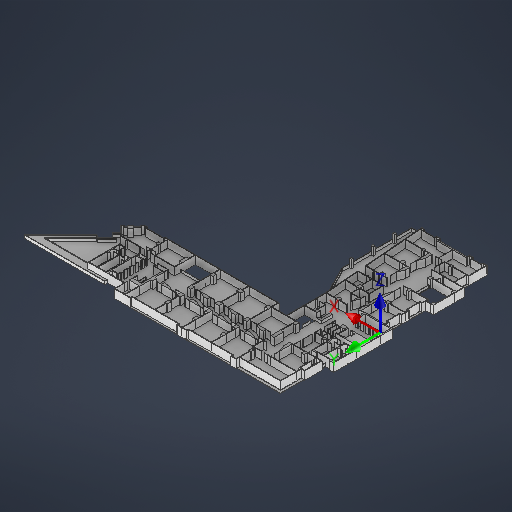
# Autodesk Inventor part: CIT-Floor-6
Saved by Autodesk Inventor 2026.1 (Build 301233020, 233B)
## iProperties
Created: 2025-08-04
Part Number: CIT-Floor-6
Material: Generic
Document SubType Name: Modeling
Designer: diego
Density: 1 g/cm^3
Appearance: Default
Author: diego
Autodesk Inventor part; units mm, degrees
(part 1 of 2)
ref_plane "YZ Plane" through (0, 0, 0) normal (1, 0, 0) x (0, 1, 0)
ref_plane "XZ Plane" through (0, 0, 0) normal (0, 1, 0) x (-1, 0, 0)
ref_plane "XY Plane" through (0, 0, 0) normal (0, 0, 1) x (1, 0, 0)
sketch "Architecture" plane through (0, 0, 0) normal (0, 1, 0) x (-1, 0, 0)
  line L0 (-168175.668, 0) -> (0, 0) construction
  line L1 (0, 0) -> (0, -118792.8893) construction
  line L2 (0, -118792.8893) -> (-168175.668, -118792.8893) construction
  line L3 (-168175.668, -118792.8893) -> (-168175.668, 0) construction
  line L4 (-25977.9567, -19239.0056) -> (-38827.9567, -19239.0056) construction
  line L5 (-23543, -30793.9912) -> (-42293, -30793.9912)
  line L6 (-42293, -30793.9912) -> (-42293, -44243.9912)
  line L7 (-42293, -44243.9912) -> (-39853, -44243.9912)
  line L8 (-39853, -44243.9912) -> (-37304.8036, -46801.098)
  line L9 (-37304.8036, -46801.098) -> (-35746.456, -45248.1806)
  line L10 (-35040.5844, -45956.5204) -> (-36598.9321, -47509.4379)
  line L11 (-36598.9321, -47509.4379) -> (-36257.3538, -47852.2105)
  line L12 (-23543, -30793.9912) -> (-33652.9783, -40945.5475)
  line L13 (-33652.9783, -40945.5475) -> (-33794.1526, -40803.8796)
  line L14 (-33794.1526, -40803.8796) -> (-33935.8206, -40945.0539)
  line L15 (-33935.8206, -40945.0539) -> (-34281.6976, -40597.9673)
  line L16 (-34281.6976, -40597.9673) -> (-38106.7328, -44409.6738)
  line L17 (-38106.7328, -44409.6738) -> (-37577.3291, -44940.9287)
  line L18 (-35040.5844, -45956.5204) -> (-36812.3221, -44178.5874)
  line L19 (-42293, -30653.9912) -> (-42293, -28903.9912)
  line L20 (-37577.3291, -44940.9287) -> (-33752.294, -41129.2222)
  line L21 (-42293, -30653.9912) -> (-23205.9885, -30653.9912)
  line L22 (-18318.5941, -27753.9912) -> (-50017.455, -27753.9912)
  line L23 (-50017.455, -27753.9912) -> (-50017.455, -28903.9912)
  line L24 (-42293, -43593.9912) -> (-42573, -43593.9912)
  line L25 (-42293, -41543.9912) -> (-42573, -41543.9912)
  line L26 (-42573, -43593.9912) -> (-42573, -44243.9912)
  line L27 (-42573, -41543.9912) -> (-42573, -41363.9912)
  line L28 (-42573, -44243.9912) -> (-47323, -44243.9912)
  line L29 (-42573, -41363.9912) -> (-44583, -41363.9912)
  line L30 (-44583, -41363.9912) -> (-44583, -39763.9912)
  line L31 (-44583, -39763.9912) -> (-44433, -39763.9912)
  line L32 (-44433, -39763.9912) -> (-44433, -41133.9912)
  line L33 (-44583, -38763.9912) -> (-44583, -38623.9912)
  line L34 (-44583, -38623.9912) -> (-43788.5906, -38623.9912)
  line L35 (-44583, -38763.9912) -> (-42573, -38763.9912)
  line L36 (-44433, -41133.9912) -> (-42573, -41133.9912)
  line L37 (-42573, -41133.9912) -> (-42573, -38763.9912)
  line L38 (-42573, -36263.9912) -> (-42573, -29203.9912)
  line L39 (-43788.5906, -37583.9912) -> (-48088.5906, -37583.9912)
  line L40 (-48088.5906, -37583.9912) -> (-48088.5906, -37443.9912)
  line L41 (-43788.5906, -37443.9912) -> (-45798.5906, -37443.9912)
  line L42 (-45798.5906, -37443.9912) -> (-45798.5906, -29203.9912)
  line L43 (-48088.5906, -37443.9912) -> (-46078.5906, -37443.9912)
  line L44 (-46078.5906, -37443.9912) -> (-46078.5906, -29203.9912)
  line L45 (-43788.5906, -36403.9912) -> (-43788.5906, -36263.9912)
  line L46 (-43788.5906, -36263.9912) -> (-42573, -36263.9912)
  line L47 (-43788.5906, -36403.9912) -> (-43788.5906, -36403.9912)
  line L48 (-42293, -28903.9912) -> (-49867.455, -28903.9912)
  line L49 (-18667.455, -27903.9912) -> (-49867.455, -27903.9912)
  line L50 (-49867.455, -27903.9912) -> (-49867.455, -28903.9912)
  line L51 (-23205.9885, -30653.9912) -> (-33554.1556, -41044.7158)
  line L52 (-33554.1556, -41044.7158) -> (-32707.1097, -41894.7236)
  line L53 (-33752.294, -41129.2222) -> (-32749.9556, -42135.0655)
  line L54 (-32749.9556, -42135.0655) -> (-18318.5941, -27753.9912)
  line L55 (-32707.1097, -41894.7236) -> (-18667.455, -27903.9912)
  line L56 (-47033, -38763.9912) -> (-49453, -38763.9912)
  line L57 (-47033, -38763.9912) -> (-47033, -38623.9912)
  line L58 (-47033, -38623.9912) -> (-48088.5906, -38623.9912)
  line L59 (-48088.5906, -36403.9912) -> (-48088.5906, -36263.9912)
  line L60 (-48088.5906, -36263.9912) -> (-49453, -36263.9912)
  line L61 (-43788.5906, -37583.9912) -> (-43788.5906, -37443.9912)
  line L62 (-49453, -29203.9912) -> (-49453, -36263.9912)
  line L63 (-49453, -38763.9912) -> (-49453, -42193.9912)
  arc A0 (-43788.5906, -38623.9912) -> (-43788.5906, -36403.9912) centre (-43788.5906, -37513.9912) ccw
  line L64 (-49453, -42193.9912) -> (-52313, -42193.9912)
  line L65 (-47323, -44243.9912) -> (-47323, -44318.9912)
  line L66 (-47323, -44318.9912) -> (-49023, -44318.9912)
  line L67 (-49023, -44318.9912) -> (-49023, -44418.9912)
  line L68 (-49023, -44418.9912) -> (-47323, -44418.9912)
  line L69 (-47323, -44418.9912) -> (-47323, -44493.9912)
  line L70 (-50223, -45658.9912) -> (-50223, -44243.9912)
  line L71 (-50223, -44243.9912) -> (-50323, -44243.9912)
  line L72 (-50323, -44243.9912) -> (-50323, -45658.9912)
  line L73 (-47323, -44493.9912) -> (-39985, -44493.9912)
  line L74 (-39985, -44493.9912) -> (-36625.0513, -47865.6888)
  line L75 (-50223, -45658.9912) -> (-48423, -45658.9912)
  line L76 (-48423, -45658.9912) -> (-48423, -45758.9912)
  line L77 (-48423, -45758.9912) -> (-50223, -45758.9912)
  line L78 (-51523, -44318.9912) -> (-51523, -44418.9912)
  line L79 (-51523, -44418.9912) -> (-53223, -44418.9912)
  line L80 (-53223, -44418.9912) -> (-53223, -44493.9912)
  line L81 (-53223, -44493.9912) -> (-60843, -44493.9912)
  line L82 (-51523, -44318.9912) -> (-53223, -44318.9912)
  line L83 (-53223, -44318.9912) -> (-53223, -44243.9912)
  line L84 (-53223, -44243.9912) -> (-61093, -44243.9912)
  line L85 (-50323, -45658.9912) -> (-52123, -45658.9912)
  line L86 (-52123, -45658.9912) -> (-52123, -45758.9912)
  line L87 (-52123, -45758.9912) -> (-50323, -45758.9912)
  line L88 (-50323, -45758.9912) -> (-50323, -52377.8595)
  line L89 (-52313, -42193.9912) -> (-52313, -41883.9912)
  line L90 (-52313, -41883.9912) -> (-52163, -41883.9912)
  line L91 (-52163, -41883.9912) -> (-52163, -42042.9956)
  line L92 (-52163, -42042.9956) -> (-49603, -42042.9956)
  line L93 (-49603, -42042.9956) -> (-49603, -40973.9912)
  line L94 (-49603, -40973.9912) -> (-52313, -40973.9912)
  line L95 (-52313, -40973.9912) -> (-52313, -39823.9912)
  line L96 (-52313, -39823.9912) -> (-52113, -39823.9912)
  line L97 (-52113, -39823.9912) -> (-52113, -40474.0396)
  line L98 (-52113, -40474.0396) -> (-49603, -40474.0396)
  line L99 (-49603, -40474.0396) -> (-49603, -30963.9912)
  line L100 (-52313, -38803.9912) -> (-52313, -37793.9912)
  line L101 (-52313, -37793.9912) -> (-52113, -37793.9912)
  line L102 (-52113, -37793.9912) -> (-52113, -38803.9912)
  line L103 (-52113, -38803.9912) -> (-52313, -38803.9912)
  line L104 (-52113, -36773.9912) -> (-52313, -36773.9912)
  line L105 (-52313, -36773.9912) -> (-52313, -35493.9912)
  line L106 (-52313, -35493.9912) -> (-52113, -35493.9912)
  line L107 (-52113, -35493.9912) -> (-52113, -36773.9912)
  line L108 (-52113, -33153.9912) -> (-52313, -33153.9912)
  line L109 (-52313, -33153.9912) -> (-52313, -34473.9912)
  line L110 (-52313, -34473.9912) -> (-52113, -34473.9912)
  line L111 (-52113, -34473.9912) -> (-52113, -33153.9912)
  line L112 (-52113, -32133.9912) -> (-52313, -32133.9912)
  line L113 (-52313, -32133.9912) -> (-52313, -31613.9912)
  line L114 (-52113, -30963.9912) -> (-52113, -32133.9912)
  line L115 (-52313, -31613.9912) -> (-52373, -31613.9912)
  line L116 (-52373, -31613.9912) -> (-52373, -30963.9912)
  line L117 (-52373, -30963.9912) -> (-52313, -30963.9912)
  line L118 (-52313, -30963.9912) -> (-52313, -30163.9912)
  line L119 (-52313, -30163.9912) -> (-52163, -30163.9912)
  line L120 (-52163, -30163.9912) -> (-52163, -30663.9912)
  line L121 (-52163, -29203.9912) -> (-50078, -29203.9912)
  line L122 (-52163, -29203.9912) -> (-52163, -29253.9912)
  line L123 (-52163, -29253.9912) -> (-52313, -29253.9912)
  line L124 (-52313, -29253.9912) -> (-52313, -29203.9912)
  line L125 (-52313, -29203.9912) -> (-56513, -29203.9912)
  line L126 (-50017.455, -28903.9912) -> (-56513, -28903.9912)
  line L127 (-49603, -30963.9912) -> (-52113, -30963.9912)
  line L128 (-52163, -30663.9912) -> (-50078, -30663.9912)
  line L129 (-50078, -30663.9912) -> (-50078, -29203.9912)
  line L130 (-56513, -29203.9912) -> (-56513, -30003.9912)
  line L131 (-56513, -30003.9912) -> (-56663, -30003.9912)
  line L132 (-56663, -30003.9912) -> (-56663, -25231.5979)
  line L133 (-56513, -31613.9912) -> (-56513, -33963.9912)
  line L134 (-56453, -30963.9912) -> (-56453, -31613.9912)
  line L135 (-56453, -31613.9912) -> (-56513, -31613.9912)
  line L136 (-56453, -30963.9912) -> (-56513, -30963.9912)
  line L137 (-56513, -30963.9912) -> (-56513, -30913.9912)
  line L138 (-56513, -30913.9912) -> (-60463, -30913.9912)
  line L139 (-56513, -33963.9912) -> (-56763, -33963.9912)
  line L140 (-56763, -33963.9912) -> (-56763, -32263.9912)
  line L141 (-56763, -32263.9912) -> (-60063, -32263.9912)
  line L142 (-56513, -40463.9912) -> (-56513, -41093.9912)
  line L143 (-56513, -40463.9912) -> (-60063, -40463.9912)
  line L144 (-56513, -42043.9912) -> (-56513, -42193.9912)
  line L145 (-56513, -42043.9912) -> (-60563, -42043.9912)
  line L146 (-56513, -41093.9912) -> (-56663, -41093.9912)
  line L147 (-56513, -42193.9912) -> (-60713, -42193.9912)
  line L148 (-60063, -40463.9912) -> (-60063, -32263.9912)
  line L149 (-56663, -25231.5979) -> (-60463, -25231.5979)
  line L150 (-60463, -25231.5979) -> (-60463, -30913.9912)
  line L151 (-56513, -28903.9912) -> (-56513, -24981.5979)
  line L152 (-56513, -24981.5979) -> (-104613, -24981.5979)
  line L153 (-56638, -37333.9912) -> (-58388, -37333.9912)
  line L154 (-58388, -37333.9912) -> (-58388, -37033.9912)
  line L155 (-58388, -37033.9912) -> (-60063, -37033.9912)
  line L156 (-56638, -33963.9912) -> (-56638, -37333.9912)
  line L157 (-60713, -25231.5979) -> (-62573, -25231.5979)
  line L158 (-56663, -41093.9912) -> (-56663, -40613.9912)
  line L159 (-56663, -40613.9912) -> (-60563, -40613.9912)
  line L160 (-60563, -40613.9912) -> (-60563, -42043.9912)
  line L161 (-60843, -44493.9912) -> (-60843, -47343.9912)
  line L162 (-36257.3538, -47852.2105) -> (-41049.7021, -52627.8595)
  line L163 (-41049.7021, -52627.8595) -> (-93819.593, -52627.8595)
  line L164 (-36625.0513, -47865.6888) -> (-37050.0552, -48289.2118)
  line L165 (-37050.0552, -48289.2118) -> (-37402.991, -47935.0419)
  line L166 (-37402.991, -47935.0419) -> (-38199.8733, -48729.1474)
  line L167 (-38199.8733, -48729.1474) -> (-38834.9879, -48091.812)
  line L168 (-38834.9879, -48091.812) -> (-39954.1648, -49207.0891)
  line L169 (-39954.1648, -49207.0891) -> (-39319.0503, -49844.4245)
  line L170 (-39319.0503, -49844.4245) -> (-40948.2319, -51467.9291)
  line L171 (-40948.2319, -51467.9291) -> (-40595.2961, -51822.099)
  line L172 (-40595.2961, -51822.099) -> (-41153, -52377.8595)
  line L173 (-41153, -52377.8595) -> (-41873, -52377.8595)
  line L174 (-41873, -52377.8595) -> (-41873, -51877.8595)
  line L175 (-41873, -51877.8595) -> (-49073, -51877.8595)
  line L176 (-49073, -51877.8595) -> (-49073, -52377.8595)
  line L177 (-49073, -52377.8595) -> (-50223, -52377.8595)
  line L178 (-37050.6723, -48642.7646) -> (-37438.9017, -48253.1777)
  line L179 (-37438.9017, -48253.1777) -> (-38058.699, -48870.8153)
  line L180 (-38058.699, -48870.8153) -> (-37670.4697, -49260.4023)
  line L181 (-50323, -52377.8595) -> (-60843, -52377.8595)
  line L182 (-60843, -52377.8595) -> (-60843, -49993.9912)
  line L183 (-60843, -47343.9912) -> (-59923, -47343.9912)
  line L184 (-59923, -47343.9912) -> (-59923, -49993.9912)
  line L185 (-59923, -49993.9912) -> (-60843, -49993.9912)
  line L186 (-50223, -48728.9912) -> (-49263, -48728.9912)
  line L187 (-49263, -48728.9912) -> (-49263, -49689)
  line L188 (-49263, -49689) -> (-50223, -49689)
  line L189 (-50223, -45758.9912) -> (-50223, -48728.9912)
  line L190 (-50223, -49689) -> (-50223, -52377.8595)
  line L191 (-61093, -46693.9912) -> (-70593, -46693.9912)
  line L192 (-61093, -46793.9912) -> (-70593, -46793.9912)
  line L193 (-61093, -44243.9912) -> (-61093, -46693.9912)
  line L194 (-70593, -46693.9912) -> (-70593, -43483.9912)
  line L195 (-70593, -43483.9912) -> (-70443, -43483.9912)
  line L196 (-70443, -43483.9912) -> (-70443, -39883.9912)
  line L197 (-70443, -39883.9912) -> (-71793, -39883.9912)
  line L198 (-46078.5906, -29203.9912) -> (-49453, -29203.9912)
  line L199 (-45798.5906, -29203.9912) -> (-42573, -29203.9912)
  line L200 (-60713, -36893.9912) -> (-61393, -36893.9912)
  line L201 (-61393, -36893.9912) -> (-61393, -35293.9912)
  line L202 (-62613, -35843.9912) -> (-64413, -35843.9912)
  line L203 (-64413, -35843.9912) -> (-64413, -36893.9912)
  line L204 (-64413, -36893.9912) -> (-65813, -36893.9912)
  line L205 (-62613, -35843.9912) -> (-62613, -35743.9912)
  line L206 (-62613, -35743.9912) -> (-69991.4271, -35743.9912)
  line L207 (-61393, -35293.9912) -> (-60713, -35293.9912)
  line L208 (-60713, -42193.9912) -> (-60713, -36893.9912)
  line L209 (-60713, -35293.9912) -> (-60713, -25231.5979)
  arc A1 (-48088.5906, -36403.9912) -> (-48088.5906, -38623.9912) centre (-48088.5906, -37513.9912) ccw
  line L210 (-48088.5906, -36403.9912) -> (-48088.5906, -36403.9912)
  line L211 (-65813, -36893.9912) -> (-68641.4271, -35893.9912)
  line L212 (-68641.4271, -35893.9912) -> (-69991.4271, -35893.9912)
  line L213 (-69991.4271, -35893.9912) -> (-69991.4271, -35743.9912)
  line L214 (-70991.4271, -36793.9912) -> (-70991.4271, -35293.9912)
  line L215 (-71552.2136, -31781.5979) -> (-71102.2136, -31781.5979)
  line L216 (-71102.2136, -31781.5979) -> (-71102.2136, -30431.5979)
  line L217 (-71102.2136, -30431.5979) -> (-71552.2136, -30431.5979)
  line L218 (-71552.2136, -30431.5979) -> (-71552.2136, -25931.5979)
  line L219 (-62573, -25231.5979) -> (-62573, -25931.5979)
  line L220 (-62573, -25931.5979) -> (-71552.2136, -25931.5979)
  line L221 (-70991.4271, -36793.9912) -> (-68963, -36793.9912)
  line L222 (-68963, -36793.9912) -> (-68963, -36893.9912)
  line L223 (-68963, -36893.9912) -> (-72363, -36893.9912)
  line L224 (-72363, -36893.9912) -> (-72363, -35293.9912)
  line L225 (-71802.2136, -31781.5979) -> (-72252.2136, -31781.5979)
  line L226 (-72252.2136, -31781.5979) -> (-72252.2136, -30431.5979)
  line L227 (-71793, -39883.9912) -> (-71793, -41493.512)
  line L228 (-71793, -41493.512) -> (-70843, -41493.512)
  line L229 (-72793, -40903.9912) -> (-74443, -40903.9912)
  line L230 (-74443, -40903.9912) -> (-76856.2965, -39883.9912)
  line L231 (-72793, -40903.9912) -> (-72793, -41053.9912)
  line L232 (-72793, -41053.9912) -> (-80086.2965, -41053.9912)
  line L233 (-76856.2965, -39883.9912) -> (-78306.2965, -39883.9912)
  line L234 (-70843, -41493.512) -> (-70843, -48653.512)
  line L235 (-70843, -48653.512) -> (-71793, -48653.512)
  line L236 (-71793, -48653.512) -> (-71793, -49993.9912)
  line L237 (-71793, -49993.9912) -> (-70843, -49993.9912)
  line L238 (-70593, -46793.9912) -> (-70593, -52377.8595)
  line L239 (-61093, -46793.9912) -> (-61093, -52377.8595)
  line L240 (-61093, -52377.8595) -> (-70593, -52377.8595)
  line L241 (-70843, -49993.9912) -> (-70843, -52377.8595)
  line L242 (-70843, -52377.8595) -> (-81981.2965, -52377.8595)
  line L243 (-80086.2965, -41053.9912) -> (-80086.2965, -40953.9912)
  line L244 (-80086.2965, -40953.9912) -> (-78306.2965, -40953.9912)
  line L245 (-78306.2965, -40953.9912) -> (-78306.2965, -39883.9912)
  line L246 (-81306.2965, -39883.9912) -> (-81306.2965, -41493.512)
  line L247 (-81306.2965, -41493.512) -> (-81981.2965, -41493.512)
  line L248 (-81981.2965, -41493.512) -> (-81981.2965, -48413.512)
  line L249 (-81981.2965, -48413.512) -> (-81306.2965, -48413.512)
  line L250 (-81306.2965, -48413.512) -> (-81306.2965, -49763.512)
  line L251 (-81306.2965, -49763.512) -> (-81981.2965, -49763.512)
  line L252 (-81306.2965, -39883.9912) -> (-82906.2965, -39883.9912)
  line L253 (-82906.2965, -39883.9912) -> (-82906.2965, -41493.512)
  line L254 (-82906.2965, -41493.512) -> (-82231.2965, -41493.512)
  line L255 (-82231.2965, -41493.512) -> (-82231.2965, -48413.512)
  line L256 (-81981.2965, -49763.512) -> (-81981.2965, -52377.8595)
  line L257 (-82231.2965, -48413.512) -> (-82906.2965, -48413.512)
  line L258 (-82906.2965, -48413.512) -> (-82906.2965, -49763.512)
  line L259 (-82906.2965, -49763.512) -> (-82231.2965, -49763.512)
  line L260 (-82231.2965, -49763.512) -> (-82231.2965, -52377.8595)
  line L261 (-82231.2965, -52377.8595) -> (-93569.593, -52377.8595)
  line L262 (-83906.2965, -40903.9912) -> (-85556.2965, -40903.9912)
  line L263 (-85556.2965, -40903.9912) -> (-87969.593, -39883.9912)
  line L264 (-83906.2965, -40903.9912) -> (-83906.2965, -41053.9912)
  line L265 (-83906.2965, -41053.9912) -> (-91199.593, -41053.9912)
  line L266 (-87969.593, -39883.9912) -> (-89419.593, -39883.9912)
  line L267 (-91199.593, -41053.9912) -> (-91199.593, -40953.9912)
  line L268 (-91199.593, -40953.9912) -> (-89419.593, -40953.9912)
  line L269 (-89419.593, -40953.9912) -> (-89419.593, -39883.9912)
  line L270 (-92419.593, -39883.9912) -> (-92419.593, -41493.512)
  line L271 (-92419.593, -41493.512) -> (-93569.593, -41493.512)
  line L272 (-93569.593, -41493.512) -> (-93569.593, -48413.512)
  line L273 (-93569.593, -48413.512) -> (-92419.593, -48413.512)
  line L274 (-92419.593, -48413.512) -> (-92419.593, -49763.512)
  line L275 (-92419.593, -49763.512) -> (-93569.593, -49763.512)
  line L276 (-92419.593, -39883.9912) -> (-93819.593, -39883.9912)
  line L277 (-93569.593, -49763.512) -> (-93569.593, -52377.8595)
  line L278 (-93819.593, -39883.9912) -> (-93819.593, -49617.8595)
  line L279 (-93819.593, -52627.8595) -> (-93819.593, -49867.8595)
  line L280 (-93819.593, -49867.8595) -> (-99463, -49867.8595)
  line L281 (-93819.593, -49617.8595) -> (-103332.8895, -49617.8595)
  line L282 (-94819.593, -41053.9912) -> (-102112.8895, -41053.9912)
  line L283 (-102112.8895, -40953.9912) -> (-100332.8895, -40953.9912)
  line L284 (-100332.8895, -40953.9912) -> (-100332.8895, -39883.9912)
  line L285 (-96469.593, -40903.9912) -> (-98882.8895, -39883.9912)
  line L286 (-94819.593, -40903.9912) -> (-96469.593, -40903.9912)
  line L287 (-98882.8895, -39883.9912) -> (-100332.8895, -39883.9912)
  line L288 (-94819.593, -40903.9912) -> (-94819.593, -41053.9912)
  line L289 (-102112.8895, -41053.9912) -> (-102112.8895, -40953.9912)
  line L290 (-104613, -39883.9912) -> (-103332.8895, -39883.9912)
  line L291 (-103332.8895, -39883.9912) -> (-103332.8895, -49617.8595)
  line L292 (-104613, -39883.9912) -> (-104613, -43633.9912)
  line L293 (-104613, -43633.9912) -> (-103613, -43633.9912)
  line L294 (-103613, -43633.9912) -> (-103613, -48333.9912)
  line L295 (-99463, -49867.8595) -> (-99463, -65265)
  line L296 (-62823, -24981.5979) -> (-62823, -25681.5979)
  line L297 (-62823, -25681.5979) -> (-81093, -25681.5979)
  line L298 (-73583, -35843.9912) -> (-75383, -35843.9912)
  line L299 (-75383, -35843.9912) -> (-75383, -36893.9912)
  line L300 (-75383, -36893.9912) -> (-76783, -36893.9912)
  line L301 (-73583, -35843.9912) -> (-73583, -35743.9912)
  line L302 (-73583, -35743.9912) -> (-80961.4271, -35743.9912)
  line L303 (-76783, -36893.9912) -> (-79611.4271, -35893.9912)
  line L304 (-79611.4271, -35893.9912) -> (-80961.4271, -35893.9912)
  line L305 (-80961.4271, -35893.9912) -> (-80961.4271, -35743.9912)
  line L306 (-81961.4271, -36793.9912) -> (-81961.4271, -35293.9912)
  line L307 (-81961.4271, -36793.9912) -> (-79883, -36793.9912)
  line L308 (-79883, -36793.9912) -> (-79883, -36893.9912)
  line L309 (-79883, -36893.9912) -> (-83243, -36893.9912)
  line L310 (-71802.2136, -35293.9912) -> (-71802.2136, -31781.5979)
  line L311 (-71552.2136, -35293.9912) -> (-71552.2136, -31781.5979)
  line L312 (-72363, -35293.9912) -> (-71802.2136, -35293.9912)
  line L313 (-71552.2136, -35293.9912) -> (-70991.4271, -35293.9912)
  line L314 (-71802.2136, -30431.5979) -> (-71802.2136, -25931.5979)
  line L315 (-72252.2136, -30431.5979) -> (-71802.2136, -30431.5979)
  line L316 (-83243, -36893.9912) -> (-83243, -25231.5979)
  line L317 (-81961.4271, -35293.9912) -> (-82993, -35293.9912)
  line L318 (-82993, -35293.9912) -> (-82993, -31781.5979)
  line L319 (-82993, -31781.5979) -> (-82043, -31781.5979)
  line L320 (-82043, -31781.5979) -> (-82043, -30431.5979)
  line L321 (-82043, -30431.5979) -> (-82993, -30431.5979)
  line L322 (-82993, -30431.5979) -> (-82993, -25231.5979)
  line L323 (-84893, -25231.5979) -> (-84893, -25931.5979)
  line L324 (-84893, -25931.5979) -> (-93843, -25931.5979)
  line L325 (-85143, -24981.5979) -> (-85143, -25681.5979)
  line L326 (-85143, -25681.5979) -> (-102463, -25681.5979)
  line L327 (-84463, -35843.9912) -> (-84463, -35743.9912)
  line L328 (-84463, -35743.9912) -> (-91841.4271, -35743.9912)
  line L329 (-84463, -35843.9912) -> (-86263, -35843.9912)
  line L330 (-86263, -35843.9912) -> (-86263, -36893.9912)
  line L331 (-86263, -36893.9912) -> (-87663, -36893.9912)
  line L332 (-87663, -36893.9912) -> (-90491.4271, -35893.9912)
  line L333 (-90491.4271, -35893.9912) -> (-91841.4271, -35893.9912)
  line L334 (-91841.4271, -35893.9912) -> (-91841.4271, -35743.9912)
  line L335 (-92841.4271, -36793.9912) -> (-90763, -36793.9912)
  line L336 (-90763, -36893.9912) -> (-94093, -36893.9912)
  line L337 (-90763, -36793.9912) -> (-90763, -36893.9912)
  line L338 (-92841.4271, -36793.9912) -> (-92841.4271, -35293.9912)
  line L339 (-94093, -36893.9912) -> (-94093, -25931.5979)
  line L340 (-92841.4271, -35293.9912) -> (-93843, -35293.9912)
  line L341 (-93843, -35293.9912) -> (-93843, -31781.5979)
  line L342 (-93843, -31781.5979) -> (-92893, -31781.5979)
  line L343 (-92893, -31781.5979) -> (-92893, -30431.5979)
  line L344 (-92893, -30431.5979) -> (-93843, -30431.5979)
  line L345 (-93843, -30431.5979) -> (-93843, -25931.5979)
  line L346 (-95313, -35843.9912) -> (-95313, -35743.9912)
  line L347 (-95313, -35743.9912) -> (-102363, -35743.9912)
  line L348 (-95313, -35843.9912) -> (-97113, -35843.9912)
  line L349 (-97113, -35843.9912) -> (-97113, -36893.9912)
  line L350 (-97113, -36893.9912) -> (-98463, -36893.9912)
  line L351 (-98463, -36893.9912) -> (-101291.4271, -35893.9912)
  line L352 (-101291.4271, -35893.9912) -> (-102363, -35893.9912)
  line L353 (-102363, -35893.9912) -> (-102363, -35743.9912)
  line L354 (-103363, -36793.9912) -> (-101463, -36793.9912)
  line L355 (-101463, -36893.9912) -> (-104613, -36893.9912)
  line L356 (-101463, -36793.9912) -> (-101463, -36893.9912)
  line L357 (-71802.2136, -25931.5979) -> (-81343, -25931.5979)
  line L358 (-81343, -25931.5979) -> (-81343, -25231.5979)
  line L359 (-81343, -25231.5979) -> (-82993, -25231.5979)
  line L360 (-81093, -25681.5979) -> (-81093, -24981.5979)
  line L361 (-83243, -25231.5979) -> (-84893, -25231.5979)
  line L362 (-102463, -25681.5979) -> (-102463, -24981.5979)
  line L363 (-94093, -25931.5979) -> (-102713, -25931.5979)
  line L364 (-102713, -25931.5979) -> (-102713, -25231.5979)
  line L365 (-102713, -25231.5979) -> (-104363, -25231.5979)
  line L366 (-104613, -36893.9912) -> (-104613, -36743.9912)
  line L367 (-104613, -36743.9912) -> (-103613, -36743.9912)
  line L368 (-103613, -36743.9912) -> (-103613, -32793.9912)
  line L369 (-103613, -32793.9912) -> (-104613, -32793.9912)
  line L370 (-104613, -32793.9912) -> (-104613, -32718.9912)
  line L371 (-104613, -32718.9912) -> (-106953, -32718.9912)
  line L372 (-106953, -32718.9912) -> (-106953, -32618.9912)
  line L373 (-106953, -32618.9912) -> (-104613, -32618.9912)
  line L374 (-107953, -32618.9912) -> (-109293, -32618.9912)
  line L375 (-107953, -32618.9912) -> (-107953, -32718.9912)
  line L376 (-107953, -32718.9912) -> (-109293, -32718.9912)
  line L377 (-109293, -32618.9912) -> (-109293, -32543.9912)
  line L378 (-109293, -32543.9912) -> (-120563, -32543.9912)
  line L379 (-109293, -32718.9912) -> (-109293, -32793.9912)
  line L380 (-109293, -32793.9912) -> (-110293, -32793.9912)
  line L381 (-104613, -32618.9912) -> (-104613, -31788.9912)
  line L382 (-104613, -31788.9912) -> (-104963, -31788.9912)
  line L383 (-104963, -31788.9912) -> (-104963, -30438.9912)
  line L384 (-104963, -30438.9912) -> (-104613, -30438.9912)
  line L385 (-104013, -31788.9912) -> (-104013, -30438.9912)
  line L386 (-104013, -30438.9912) -> (-104363, -30438.9912)
  line L387 (-103363, -36793.9912) -> (-103363, -32543.9912)
  line L388 (-104363, -30438.9912) -> (-104363, -25231.5979)
  line L389 (-104613, -25231.5979) -> (-121713, -25231.5979)
  line L390 (-121713, -25231.5979) -> (-121713, -34443.9912)
  line L391 (-120763, -34443.9912) -> (-120763, -26252.4158)
  line L392 (-120763, -26252.4158) -> (-104613, -26252.4158)
  line L393 (-104013, -31788.9912) -> (-104363, -31788.9912)
  line L394 (-104363, -31788.9912) -> (-104363, -32543.9912)
  line L395 (-104363, -32543.9912) -> (-103363, -32543.9912)
  line L396 (-104613, -26452.4158) -> (-120563, -26452.4158)
  line L397 (-120563, -26452.4158) -> (-120563, -32543.9912)
  line L398 (-104613, -30438.9912) -> (-104613, -26452.4158)
  line L399 (-104613, -26252.4158) -> (-104613, -24981.5979)
  line L400 (-110293, -32793.9912) -> (-110293, -33093.9912)
  line L401 (-110293, -33093.9912) -> (-110393, -33093.9912)
  line L402 (-110393, -33093.9912) -> (-110393, -32793.9912)
  line L403 (-110293, -34313.9912) -> (-110293, -36483.9912)
  line L404 (-110293, -34313.9912) -> (-110393, -34313.9912)
  line L405 (-110393, -34313.9912) -> (-110393, -41098.8644)
  line L406 (-110293, -36483.9912) -> (-109293, -38948.8644)
  line L407 (-109293, -38948.8644) -> (-109293, -41348.8644)
  line L408 (-109293, -41348.8644) -> (-110843, -41348.8644)
  line L409 (-110843, -41348.8644) -> (-110843, -44048.8644)
  line L410 (-110393, -41098.8644) -> (-115263, -41098.8644)
  line L411 (-110393, -32793.9912) -> (-120563, -32793.9912)
  line L412 (-120563, -32793.9912) -> (-120563, -34443.9912)
  line L413 (-120563, -34443.9912) -> (-119833, -34443.9912)
  line L414 (-119833, -34443.9912) -> (-119833, -39213.9912)
  line L415 (-119833, -39213.9912) -> (-120083, -39213.9912)
  line L416 (-120083, -39213.9912) -> (-120083, -34693.9912)
  line L417 (-120083, -34693.9912) -> (-121763, -34693.9912)
  line L418 (-121763, -34693.9912) -> (-121763, -41098.8644)
  line L419 (-121763, -41098.8644) -> (-120083, -41098.8644)
  line L420 (-120083, -41098.8644) -> (-120083, -40118.8644)
  line L421 (-120083, -40118.8644) -> (-119833, -40118.8644)
  line L422 (-119833, -40118.8644) -> (-119833, -41098.8644)
  line L423 (-116383, -41098.8644) -> (-116383, -39883.8644)
  line L424 (-116383, -39883.8644) -> (-115263, -39883.8644)
  line L425 (-115263, -39883.8644) -> (-115263, -41098.8644)
  line L426 (-116383, -41098.8644) -> (-119833, -41098.8644)
  line L427 (-103613, -48333.9912) -> (-104613, -48333.9912)
  line L428 (-104613, -48333.9912) -> (-104613, -49867.8595)
  line L429 (-104613, -49867.8595) -> (-99713, -49867.8595)
  line L430 (-99713, -49867.8595) -> (-99713, -56717.8595)
  line L431 (-120763, -34443.9912) -> (-122013, -34443.9912)
  line L432 (-122013, -34443.9912) -> (-122013, -41348.8644)
  line L433 (-122013, -41348.8644) -> (-121533, -41348.8644)
  line L434 (-121533, -41348.8644) -> (-121533, -43318.8644)
  line L435 (-110843, -44048.8644) -> (-110943, -44048.8644)
  line L436 (-110943, -44048.8644) -> (-110943, -41348.8644)
  line L437 (-110943, -44968.8644) -> (-110943, -48548.8644)
  line L438 (-110943, -48548.8644) -> (-110843, -48548.8644)
  line L439 (-110843, -48548.8644) -> (-110843, -44968.8644)
  line L440 (-110843, -44968.8644) -> (-110943, -44968.8644)
  line L441 (-110943, -41348.8644) -> (-116463, -41348.8644)
  line L442 (-110843, -49468.8644) -> (-110843, -51968.8644)
  line L443 (-110843, -49468.8644) -> (-110943, -49468.8644)
  line L444 (-110943, -49468.8644) -> (-110943, -49618.8644)
  line L445 (-110943, -49618.8644) -> (-114343, -49618.8644)
  line L446 (-116463, -41348.8644) -> (-116463, -42028.8644)
  line L447 (-116463, -42028.8644) -> (-116563, -42028.8644)
  line L448 (-116563, -42028.8644) -> (-116563, -41348.8644)
  line L449 (-116563, -41348.8644) -> (-121383, -41348.8644)
  line L450 (-121383, -41348.8644) -> (-121383, -43318.8644)
  line L451 (-121383, -43318.8644) -> (-118123, -43318.8644)
  line L452 (-118123, -43318.8644) -> (-118123, -42928.8644)
  line L453 (-118123, -42928.8644) -> (-116323, -42928.8644)
  line L454 (-116323, -42928.8644) -> (-116323, -49618.8644)
  line L455 (-114343, -49618.8644) -> (-114343, -48728.9912)
  line L456 (-114343, -48728.9912) -> (-115323, -48728.9912)
  line L457 (-115323, -48728.9912) -> (-115323, -49618.8644)
  line L458 (-115323, -49618.8644) -> (-116323, -49618.8644)
  line L459 (-110843, -51968.8644) -> (-110993, -51968.8644)
  line L460 (-110993, -51968.8644) -> (-110993, -49838.8644)
  line L461 (-103963, -49867.8595) -> (-103963, -51867.8595)
  line L462 (-103963, -51867.8595) -> (-103813, -51867.8595)
  line L463 (-103813, -51867.8595) -> (-103813, -54717.8595)
  line L464 (-103813, -54717.8595) -> (-103963, -54717.8595)
  line L465 (-103963, -54717.8595) -> (-103963, -56717.8595)
  line L466 (-99713, -56717.8595) -> (-106343, -56717.8595)
  line L467 (-106343, -56717.8595) -> (-106343, -61217.8595)
  line L468 (-110993, -49838.8644) -> (-113662.994, -49838.8644)
  line L469 (-113662.994, -49838.8644) -> (-113662.994, -51768.8644)
  line L470 (-113662.994, -51768.8644) -> (-111913, -51768.8644)
  line L471 (-111913, -51768.8644) -> (-111913, -51968.8644)
  line L472 (-111913, -51968.8644) -> (-115063, -51968.8644)
  line L473 (-115063, -51968.8644) -> (-115063, -51768.8644)
  line L474 (-115063, -51768.8644) -> (-113882.994, -51768.8644)
  line L475 (-113882.994, -51768.8644) -> (-113882.994, -49838.8644)
  line L476 (-113882.994, -49838.8644) -> (-116212.994, -49838.8644)
  line L477 (-115983, -51768.8644) -> (-115983, -51968.8644)
  line L478 (-115983, -51968.8644) -> (-118703, -51968.8644)
  line L479 (-118703, -51968.8644) -> (-118703, -51768.8644)
  line L480 (-118703, -51768.8644) -> (-117553, -51768.8644)
  line L481 (-117553, -49068.8644) -> (-118073, -49068.8644)
  line L482 (-118073, -49068.8644) -> (-118073, -48868.8644)
  line L483 (-118073, -48868.8644) -> (-116573, -48868.8644)
  line L484 (-116573, -48868.8644) -> (-116573, -43568.8644)
  line L485 (-116573, -43568.8644) -> (-120403, -43568.8644)
  line L486 (-120403, -43568.8644) -> (-120403, -50068.8644)
  line L487 (-120403, -50068.8644) -> (-118003, -50068.8644)
  line L488 (-118003, -50068.8644) -> (-118003, -50268.8644)
  line L489 (-118003, -50268.8644) -> (-120403, -50268.8644)
  line L490 (-120403, -50268.8644) -> (-120403, -51768.8644)
  line L491 (-120403, -51768.8644) -> (-120053, -51768.8644)
  line L492 (-120053, -51768.8644) -> (-120053, -51968.8644)
  line L493 (-120053, -51968.8644) -> (-122773, -51968.8644)
  line L494 (-122773, -51968.8644) -> (-122773, -51768.8644)
  line L495 (-122773, -51768.8644) -> (-121623, -51768.8644)
  arc A2 (-117553, -51768.8644) -> (-117553, -49068.8644) centre (-117976.9399, -50418.8644) ccw
  line L496 (-115983, -51768.8644) -> (-116212.994, -51768.8644)
  line L497 (-116212.994, -51768.8644) -> (-116212.994, -49838.8644)
  line L498 (-117553, -51768.8644) -> (-117553, -49068.8644) construction
  line L499 (-121533, -43318.8644) -> (-123223, -43318.8644)
  line L500 (-123223, -43318.8644) -> (-123223, -42918.8644)
  line L501 (-123223, -42918.8644) -> (-125023, -42918.8644)
  line L502 (-125023, -42918.8644) -> (-125023, -66248.8644)
  line L503 (-123903, -43568.8644) -> (-120653, -43568.8644)
  line L504 (-120653, -43568.8644) -> (-120653, -48868.8644)
  line L505 (-120653, -48868.8644) -> (-122143, -48868.8644)
  line L506 (-122143, -48868.8644) -> (-122143, -49068.8644)
  line L507 (-122143, -49068.8644) -> (-121623, -49068.8644)
  line L508 (-121623, -49068.8644) -> (-121623, -51768.8644) construction
  arc A3 (-121623, -51768.8644) -> (-121623, -49068.8644) centre (-122046.9399, -50418.8644) ccw
  line L509 (-123903, -43568.8644) -> (-123903, -44018.8644)
  line L510 (-123903, -44018.8644) -> (-124773, -44018.8644)
  line L511 (-124773, -44018.8644) -> (-124773, -50068.8644)
  line L512 (-124773, -50068.8644) -> (-122373, -50068.8644)
  line L513 (-122373, -50068.8644) -> (-122373, -50268.8644)
  line L514 (-122373, -50268.8644) -> (-124773, -50268.8644)
  line L515 (-124773, -50268.8644) -> (-124773, -51768.8644)
  line L516 (-124773, -51768.8644) -> (-124423, -51768.8644)
  line L517 (-124423, -51768.8644) -> (-124423, -51968.8644)
  line L518 (-124423, -51968.8644) -> (-124773, -51968.8644)
  line L519 (-124773, -51968.8644) -> (-124773, -53418.8644)
  line L520 (-124773, -53418.8644) -> (-124423, -53418.8644)
  line L521 (-124423, -53418.8644) -> (-124423, -53118.8644)
  line L522 (-124423, -53118.8644) -> (-123873, -53118.8644)
  line L523 (-123873, -53118.8644) -> (-123873, -53418.8644)
  line L524 (-123873, -53418.8644) -> (-115203, -53418.8644)
  line L525 (-115203, -53418.8644) -> (-115203, -53668.8644)
  line L526 (-115203, -53668.8644) -> (-115842, -53668.8644)
  line L527 (-115842, -53668.8644) -> (-115842, -56879.3995)
  line L528 (-115842, -56879.3995) -> (-115203, -56879.3995)
  line L529 (-115203, -56879.3995) -> (-115203, -56368.8644)
  line L530 (-115203, -56368.8644) -> (-114283, -56368.8644)
  line L531 (-114283, -56368.8644) -> (-114283, -53418.8644)
  line L532 (-114283, -53418.8644) -> (-114033, -53418.8644)
  line L533 (-114033, -53418.8644) -> (-114033, -56368.8644)
  line L534 (-114033, -56368.8644) -> (-112663, -56368.8644)
  line L535 (-112663, -56368.8644) -> (-112663, -53668.8644)
  line L536 (-112663, -53668.8644) -> (-113113, -53668.8644)
  line L537 (-113113, -53668.8644) -> (-113113, -53418.8644)
  line L538 (-113113, -53418.8644) -> (-111913, -53418.8644)
  line L539 (-110843, -53418.8644) -> (-110843, -57818.8644)
  line L540 (-110843, -53418.8644) -> (-110993, -53418.8644)
  line L541 (-110993, -53418.8644) -> (-110993, -56368.8644)
  line L542 (-111913, -53418.8644) -> (-111913, -53668.8644)
  line L543 (-111913, -53668.8644) -> (-112413, -53668.8644)
  line L544 (-112413, -53668.8644) -> (-112413, -56368.8644)
  line L545 (-112413, -56368.8644) -> (-110993, -56368.8644)
  line L546 (-110843, -57818.8644) -> (-110993, -57818.8644)
  line L547 (-110993, -57818.8644) -> (-110993, -56618.8644)
  line L548 (-110993, -56618.8644) -> (-113793, -56618.8644)
  line L549 (-113793, -56618.8644) -> (-113793, -57818.8644)
  line L550 (-113793, -57818.8644) -> (-115293, -57818.8644)
  line L551 (-104613, -56717.8595) -> (-104613, -58117.8595)
  line L552 (-106343, -61217.8595) -> (-105363, -61217.8595)
  line L553 (-105363, -61217.8595) -> (-105363, -57577.8595)
  line L554 (-105363, -57577.8595) -> (-104613, -57577.8595)
  line L555 (-104213, -58117.8595) -> (-104213, -61217.8595)
  line L556 (-104213, -61217.8595) -> (-103663, -61217.8595)
  line L557 (-103663, -61217.8595) -> (-101213, -61217.8595)
  line L558 (-101213, -61217.8595) -> (-101213, -61117.8595)
  line L559 (-101213, -61117.8595) -> (-103563, -61117.8595)
  line L560 (-103563, -61117.8595) -> (-103563, -58117.8595)
  line L561 (-103663, -61217.8595) -> (-103663, -58117.8595)
  line L562 (-103463, -58117.8595) -> (-103463, -56967.8595)
  line L563 (-103463, -56967.8595) -> (-99713, -56967.8595)
  line L564 (-100313, -61217.8595) -> (-99713, -61217.8595)
  line L565 (-100313, -61217.8595) -> (-100313, -61117.8595)
  line L566 (-100313, -61117.8595) -> (-99713, -61117.8595)
  line L567 (-99713, -56967.8595) -> (-99713, -61117.8595)
  line L568 (-99713, -61217.8595) -> (-99713, -65217.8595)
  line L569 (-100263, -61217.8595) -> (-100263, -62617.8595)
  line L570 (-100263, -62617.8595) -> (-99713, -62617.8595)
  line L571 (-99713, -65217.8595) -> (-103563, -65217.8595)
  line L572 (-103563, -65217.8595) -> (-103563, -65067.8595)
  line L573 (-103563, -65067.8595) -> (-104713, -65067.8595)
  line L574 (-104713, -65067.8595) -> (-104713, -65217.8595)
  line L575 (-104713, -65217.8595) -> (-107613, -65217.8595)
  line L576 (-107613, -65217.8595) -> (-107613, -65817.8595)
  line L577 (-104613, -58117.8595) -> (-103663, -58117.8595)
  line L578 (-103563, -58117.8595) -> (-103463, -58117.8595)
  line L579 (-114023, -62318.8644) -> (-115133, -62318.8644)
  line L580 (-114023, -62318.8644) -> (-114023, -65018.8644)
  line L581 (-114023, -65018.8644) -> (-113723, -65018.8644)
  line L582 (-113723, -65018.8644) -> (-113723, -65998.8644)
  line L583 (-113723, -65998.8644) -> (-111623, -65998.8644)
  line L584 (-111623, -65998.8644) -> (-111623, -67868.8644)
  line L585 (-115293, -57818.8644) -> (-115293, -57568.8644)
  line L586 (-115293, -57568.8644) -> (-116143, -57568.8644)
  line L587 (-116143, -57568.8644) -> (-116143, -53691.819)
  line L588 (-117293, -57568.8644) -> (-123873, -57568.8644)
  line L589 (-117293, -57568.8644) -> (-117293, -57268.8644)
  line L590 (-117293, -57268.8644) -> (-118223, -57268.8644)
  line L591 (-116143, -53691.819) -> (-118223, -53691.819)
  line L592 (-118223, -53691.819) -> (-118223, -53991.819)
  line L593 (-118223, -53991.819) -> (-122278, -53991.819)
  line L594 (-118223, -57268.8644) -> (-118223, -56968.8644)
  line L595 (-118223, -56968.8644) -> (-121883, -56968.8644)
  line L596 (-118823, -53991.819) -> (-118823, -55480.3417)
  line L597 (-118823, -55480.3417) -> (-119323, -55480.3417)
  line L598 (-119323, -55480.3417) -> (-119323, -56968.8644)
  line L599 (-123873, -57568.8644) -> (-123873, -57868.8644)
  line L600 (-123873, -57868.8644) -> (-124423, -57868.8644)
  line L601 (-124423, -57868.8644) -> (-124423, -57818.8644)
  line L602 (-124423, -57818.8644) -> (-124773, -57818.8644)
  line L603 (-124773, -57818.8644) -> (-124773, -61418.8644)
  line L604 (-124773, -61418.8644) -> (-124423, -61418.8644)
  line L605 (-124423, -61418.8644) -> (-124423, -61368.8644)
  line L606 (-124423, -61368.8644) -> (-123873, -61368.8644)
  line L607 (-123873, -61368.8644) -> (-123873, -62318.8644)
  line L608 (-115133, -62318.8644) -> (-115133, -62618.8644)
  line L609 (-115133, -62618.8644) -> (-114523, -62618.8644)
  line L610 (-116083, -62318.8644) -> (-117233, -62318.8644)
  line L611 (-117233, -62318.8644) -> (-117233, -62618.8644)
  line L612 (-117233, -62618.8644) -> (-116083, -62618.8644)
  line L613 (-116083, -62618.8644) -> (-116083, -62318.8644)
  line L614 (-123873, -62318.8644) -> (-122273, -62318.8644)
  line L615 (-122273, -62318.8644) -> (-122273, -62618.8644)
  line L616 (-122273, -62618.8644) -> (-124523, -62618.8644)
  line L617 (-121023, -62618.8644) -> (-121023, -62318.8644)
  line L618 (-121023, -62318.8644) -> (-120273, -62318.8644)
  line L619 (-120273, -62318.8644) -> (-120273, -62618.8644)
  line L620 (-120273, -62618.8644) -> (-121023, -62618.8644)
  line L621 (-119323, -62618.8644) -> (-119323, -62318.8644)
  line L622 (-119323, -62318.8644) -> (-118183, -62318.8644)
  line L623 (-118183, -62318.8644) -> (-118183, -62618.8644)
  line L624 (-118183, -62618.8644) -> (-119323, -62618.8644)
  line L625 (-124523, -62618.8644) -> (-124523, -65748.8644)
  line L626 (-124523, -65748.8644) -> (-114523, -65748.8644)
  line L627 (-114523, -65748.8644) -> (-114523, -62618.8644)
  line L628 (-111623, -67868.8644) -> (-112423, -70374.2386)
  line L629 (-112423, -70374.2386) -> (-112423, -72774.2386)
  line L630 (-111623, -74024.2386) -> (-114503, -74024.2386)
  line L631 (-112423, -72774.2386) -> (-112523, -72774.2386)
  line L632 (-112523, -72774.2386) -> (-112523, -66248.8644)
  line L633 (-112523, -66248.8644) -> (-121793, -66248.8644)
  line L634 (-111623, -74024.2386) -> (-111623, -76754.2386)
  line L635 (-125023, -66248.8644) -> (-122043, -66248.8644)
  line L636 (-122043, -66248.8644) -> (-122043, -82109.6129)
  line L637 (-122043, -67698.8644) -> (-121313, -67698.8644)
  line L638 (-121313, -67698.8644) -> (-121313, -72574.2386)
  line L639 (-121313, -72574.2386) -> (-122043, -72574.2386)
  line L640 (-121793, -66248.8644) -> (-121793, -67448.8644)
  line L641 (-121793, -67448.8644) -> (-121093, -67448.8644)
  line L642 (-121093, -67448.8644) -> (-121093, -72824.2386)
  line L643 (-121093, -72824.2386) -> (-121793, -72824.2386)
  line L644 (-121793, -72824.2386) -> (-121793, -74024.2386)
  line L645 (-121793, -74024.2386) -> (-115613, -74024.2386)
  line L646 (-115613, -74024.2386) -> (-115613, -73554.2386)
  line L647 (-115613, -73554.2386) -> (-114503, -73554.2386)
  line L648 (-114503, -73554.2386) -> (-114503, -74024.2386)
  line L649 (-111623, -76754.2386) -> (-112423, -79259.6129)
  line L650 (-112423, -79259.6129) -> (-112423, -81659.6129)
  line L651 (-112423, -81659.6129) -> (-112523, -81659.6129)
  line L652 (-112523, -81659.6129) -> (-112523, -74224.2386)
  line L653 (-112523, -74224.2386) -> (-114503, -74224.2386)
  line L654 (-114503, -74224.2386) -> (-114503, -74924.2386)
  line L655 (-114503, -74924.2386) -> (-115613, -74924.2386)
  line L656 (-115613, -74924.2386) -> (-115613, -74224.2386)
  line L657 (-115613, -74224.2386) -> (-121793, -74224.2386)
  line L658 (-121793, -74224.2386) -> (-121793, -75424.2386)
  line L659 (-121793, -75424.2386) -> (-121093, -75424.2386)
  line L660 (-121093, -75424.2386) -> (-121093, -80799.6129)
  line L661 (-112423, -82909.6129) -> (-114503, -82909.6129)
  line L662 (-112423, -82909.6129) -> (-112423, -83059.6129)
  line L663 (-112423, -83059.6129) -> (-114503, -83059.6129)
  line L664 (-114503, -82909.6129) -> (-114503, -81959.6129)
  line L665 (-114503, -81959.6129) -> (-115613, -81959.6129)
  line L666 (-115613, -81959.6129) -> (-115613, -82909.6129)
  line L667 (-115613, -82909.6129) -> (-121793, -82909.6129)
  line L668 (-114503, -83059.6129) -> (-114503, -83259.6129)
  line L669 (-115613, -83259.6129) -> (-115613, -83159.6129)
  line L670 (-115613, -83159.6129) -> (-122043, -83159.6129)
  line L671 (-121093, -80799.6129) -> (-121793, -80799.6129)
  line L672 (-121793, -80799.6129) -> (-121793, -82909.6129)
  line L673 (-115103, -83259.6129) -> (-115103, -90309.6129)
  line L674 (-70593, -46793.9912) -> (-70593, -46693.9912)
  line L675 (-61093, -46793.9912) -> (-61093, -46693.9912)
  line L676 (-122043, -80549.6129) -> (-121313, -80549.6129)
  line L677 (-121313, -80549.6129) -> (-121313, -75674.2386)
  line L678 (-121313, -75674.2386) -> (-122043, -75674.2386)
  line L679 (-122043, -82109.6129) -> (-125023, -82109.6129)
  line L680 (-125023, -82109.6129) -> (-125023, -94209.6129)
  line L681 (-122043, -83159.6129) -> (-122043, -82359.6129)
  line L682 (-122043, -82359.6129) -> (-123873, -82359.6129)
  line L683 (-123873, -82359.6129) -> (-123873, -83259.6129)
  line L684 (-123873, -83259.6129) -> (-124773, -83259.6129)
  line L685 (-124773, -83259.6129) -> (-124773, -90569.6129)
  line L686 (-115203, -83259.6129) -> (-115203, -90309.6129)
  line L687 (-115103, -90309.6129) -> (-114503, -90309.6129)
  line L688 (-114503, -90309.6129) -> (-114503, -91609.6129)
  line L689 (-115203, -90309.6129) -> (-115613, -90309.6129)
  line L690 (-114503, -83259.6129) -> (-115103, -83259.6129)
  line L691 (-115203, -83259.6129) -> (-115613, -83259.6129)
  line L692 (-115203, -83259.6129) -> (-115103, -83259.6129)
  line L693 (-115103, -90309.6129) -> (-115203, -90309.6129)
  line L694 (-114503, -91609.6129) -> (-115613, -91609.6129)
  line L695 (-115613, -90309.6129) -> (-115613, -91059.6129)
  line L696 (-115613, -91059.6129) -> (-123873, -91059.6129)
  line L697 (-115613, -91609.6129) -> (-115613, -91309.6129)
  line L698 (-115613, -91309.6129) -> (-116963, -91309.6129)
  line L699 (-116963, -91309.6129) -> (-116963, -92809.6129)
  line L700 (-116963, -92809.6129) -> (-117113, -92809.6129)
  line L701 (-117113, -92809.6129) -> (-117113, -91309.6129)
  line L702 (-116963, -93959.6129) -> (-116963, -94009.6129)
  line L703 (-116963, -94009.6129) -> (-112303, -94009.6129)
  line L704 (-116963, -93959.6129) -> (-124773, -93959.6129)
  line L705 (-117113, -91309.6129) -> (-123873, -91309.6129)
  line L706 (-124773, -90569.6129) -> (-123873, -90569.6129)
  line L707 (-123873, -90569.6129) -> (-123873, -91059.6129)
  line L708 (-123873, -91309.6129) -> (-123873, -91529.6129)
  line L709 (-123873, -91529.6129) -> (-124773, -91529.6129)
  line L710 (-124773, -91529.6129) -> (-124773, -93959.6129)
  line L711 (-122043, -94209.6129) -> (-122043, -106379.6129)
  line L712 (-122043, -106379.6129) -> (-115043, -106379.6129)
  line L713 (-120923, -93959.6129) -> (-120923, -92634.6129)
  line L714 (-120923, -92634.6129) -> (-120323, -92634.6129)
  line L715 (-120323, -92634.6129) -> (-120323, -91309.6129)
  line L716 (-112303, -94009.6129) -> (-112303, -94159.6129)
  line L717 (-121313, -94209.6129) -> (-125023, -94209.6129)
  line L718 (-112303, -95379.6129) -> (-112403, -95379.6129)
  line L719 (-121313, -94209.6129) -> (-121313, -99029.6129)
  line L720 (-112303, -95379.6129) -> (-112303, -99279.6129)
  line L721 (-112403, -95379.6129) -> (-112403, -97149.6129)
  line L722 (-112403, -97149.6129) -> (-112453, -97149.6129)
  line L723 (-112453, -97149.6129) -> (-112453, -99029.6129)
  line L724 (-112303, -99279.6129) -> (-114603, -99279.6129)
  line L725 (-112453, -99029.6129) -> (-114603, -99029.6129)
  line L726 (-114603, -99029.6129) -> (-114603, -98659.6129)
  line L727 (-114603, -98659.6129) -> (-115568, -98659.6129)
  line L728 (-115568, -98659.6129) -> (-115568, -99029.6129)
  line L729 (-114603, -99279.6129) -> (-114603, -99649.6129)
  line L730 (-114603, -99649.6129) -> (-115568, -99649.6129)
  line L731 (-115568, -99649.6129) -> (-115568, -99279.6129)
  line L732 (-115568, -99279.6129) -> (-121793, -99279.6129)
  line L733 (-121793, -99279.6129) -> (-121793, -106129.6129)
  line L734 (-111083, -99179.6129) -> (-108683, -99179.6129)
  line L735 (-111083, -99179.6129) -> (-111083, -99279.6129)
  line L736 (-111083, -99279.6129) -> (-109933, -99279.6129)
  line L737 (-112303, -94159.6129) -> (-116963, -94159.6129)
  line L738 (-121113, -94209.6129) -> (-116963, -94209.6129)
  line L739 (-116963, -94209.6129) -> (-116963, -94159.6129)
  line L740 (-109933, -99279.6129) -> (-109933, -104849.6129)
  line L741 (-109833, -99279.6129) -> (-109833, -104849.6129)
  line L742 (-109833, -99279.6129) -> (-108683, -99279.6129)
  line L743 (-108683, -99279.6129) -> (-108683, -99179.6129)
  line L744 (-121793, -106129.6129) -> (-120593, -106129.6129)
  line L745 (-120593, -106129.6129) -> (-120593, -105439.6129)
  line L746 (-120593, -105439.6129) -> (-116493, -105439.6129)
  line L747 (-116493, -105439.6129) -> (-116493, -106129.6129)
  line L748 (-116493, -106129.6129) -> (-115293, -106129.6129)
  line L749 (-115293, -106129.6129) -> (-115293, -104849.6129)
  line L750 (-115043, -106379.6129) -> (-115043, -105429.6129)
  line L751 (-115043, -105429.6129) -> (-103743, -105429.6129)
  line L752 (-120343, -106379.6129) -> (-120343, -105639.6129)
  line L753 (-120343, -105639.6129) -> (-116743, -105639.6129)
  line L754 (-116743, -105639.6129) -> (-116743, -106379.6129)
  line L755 (-115293, -104849.6129) -> (-109933, -104849.6129)
  line L756 (-121113, -94209.6129) -> (-121113, -99029.6129)
  line L757 (-115568, -99029.6129) -> (-121113, -99029.6129)
  line L758 (-121313, -99029.6129) -> (-122043, -99029.6129)
  line L759 (-109833, -104849.6129) -> (-103493, -104849.6129)
  line L760 (-103743, -105429.6129) -> (-103743, -106379.6129)
  line L761 (-103743, -106379.6129) -> (-96202.3887, -106379.6129)
  line L762 (-103493, -104849.6129) -> (-103493, -106129.6129)
  line L763 (-103493, -106129.6129) -> (-102293, -106129.6129)
  line L764 (-102293, -106129.6129) -> (-102293, -105439.6129)
  line L765 (-102293, -105439.6129) -> (-97223, -105439.6129)
  line L766 (-96202.3887, -106379.6129) -> (-99463, -65265)
  line L767 (-97223, -105439.6129) -> (-97223, -106129.6129)
  line L768 (-97223, -106129.6129) -> (-96473, -106129.6129)
  line L769 (-96473, -106129.6129) -> (-97016.2421, -99279.6129)
  line L770 (-102043, -106379.6129) -> (-102043, -105639.6129)
  line L771 (-102043, -105639.6129) -> (-97473, -105639.6129)
  line L772 (-97473, -105639.6129) -> (-97473, -106379.6129)
  line L773 (-107403, -99179.6129) -> (-107403, -96479.6129)
  line L774 (-107463, -99179.6129) -> (-107463, -99279.6129)
  line L775 (-107463, -99279.6129) -> (-104613, -99279.6129)
  line L776 (-107403, -96479.6129) -> (-106453, -94037.9126)
  line L777 (-106453, -94037.9126) -> (-106453, -91637.9126)
  line L778 (-104613, -99279.6129) -> (-104613, -99649.6129)
  line L779 (-104613, -99649.6129) -> (-103653, -99649.6129)
  line L780 (-103653, -99649.6129) -> (-103653, -99279.6129)
  line L781 (-103653, -99279.6129) -> (-97016.2421, -99279.6129)
  line L782 (-106453, -91637.9126) -> (-106353, -91637.9126)
  line L783 (-106353, -91637.9126) -> (-106353, -99029.6129)
  line L784 (-107463, -99179.6129) -> (-107403, -99179.6129)
  line L785 (-104713, -90417.9126) -> (-107403, -90417.9126)
  line L786 (-107403, -90417.9126) -> (-107403, -88767.9126)
  line L787 (-104713, -90417.9126) -> (-104713, -91617.9126)
  line L788 (-104713, -91617.9126) -> (-103563, -91617.9126)
  line L789 (-103563, -91617.9126) -> (-103563, -90417.9126)
  line L790 (-103563, -90417.9126) -> (-97719.0229, -90417.9126)
  line L791 (-97036.0684, -99029.6129) -> (-97719.0229, -90417.9126)
  line L792 (-107403, -88767.9126) -> (-106453, -86326.2124)